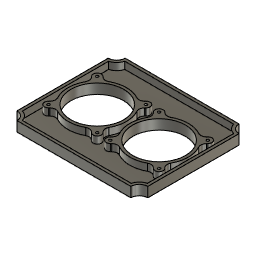
internal_frame (Autodesk Fusion 360 design; units mm, degrees)
Autodesk Fusion 360 part; units mm, degrees
note: some values were not read from the file. Set by a fixed rule: which face or edge a step refers to.
sketch "Sketch1" plane through (0, 0, 0) normal (0, 0, 1) x (1, 0, 0)
  line L0 (69.35, 57.35) -> (-69.35, 57.35)
  line L1 (-69.35, 57.35) -> (-69.35, -57.35)
  line L2 (-69.35, -57.35) -> (69.35, -57.35)
  line L3 (69.35, -57.35) -> (69.35, 57.35)
  line L4 (69.35, 57.35) -> (-69.35, -57.35) construction
  line L5 (-69.35, 57.35) -> (69.35, -57.35) construction
  circle A0 centre (-69.35, -57.35) radius 9
  circle A1 centre (-69.35, 57.35) radius 9
  circle A2 centre (69.35, 57.35) radius 9
  circle A3 centre (69.35, -57.35) radius 9
  line L6 (-69.35, 0) -> (69.35, 0) construction
  line L7 (0, 57.35) -> (0, -57.35) construction
  dimension "d1" = 138.7
  dimension "d2" = 114.7
  dimension "d3" = 18
  dimension "d4" = 18
  dimension "d5" = 18
  dimension "d6" = 18
  constraint horizontal L0
  constraint perpendicular L0 L1
  constraint parallel L0 L2
  constraint parallel L1 L3
  constraint coincident L4 origin
  constraint coincident L5 origin
  constraint coincident L1.end L2.start
  constraint coincident L0.end L1.start
  constraint coincident L0.start L3.end
  constraint coincident L2.end L3.start
  constraint midpoint L1 L6.start
  constraint midpoint L3 L6.end
  constraint midpoint L0 L7.start
  constraint midpoint L2 L7.end
  measures "d1" distance of L1 L3
  measures "d2" distance of L0 L2
  measures "d3" diameter of A0
  measures "d4" diameter of A1
  measures "d5" diameter of A2
  measures "d6" diameter of A3
extrude "Extrude1" add sketch "Sketch1" along normal blind 10.5 contours L0 L1 L2 L3 A0 A1 A2 A3
sketch "Sketch2" plane through (0, 0, 10.5) normal (0, 0, 1) x (-1, 0, 0)
  line L0 (69.35, -48.35) -> (69.35, 48.35)
  arc A0 (60.35, 57.35) -> (69.35, 48.35) centre (69.35, 57.35) ccw
  line L1 (60.35, 57.35) -> (-60.35, 57.35)
  arc A1 (-69.35, 48.35) -> (-60.35, 57.35) centre (-69.35, 57.35) ccw
  line L2 (-69.35, 48.35) -> (-69.35, -48.35)
  arc A2 (-60.35, -57.35) -> (-69.35, -48.35) centre (-69.35, -57.35) ccw
  line L3 (-60.35, -57.35) -> (60.35, -57.35)
  arc A3 (69.35, -48.35) -> (60.35, -57.35) centre (69.35, -57.35) ccw
  line L4 (69.35, 0) -> (-69.8, 0) construction
  line L5 (0, -57.35) -> (0, 57.35) construction
  circle A4 centre (32.6, 0) radius 28
  circle A5 centre (-33, 0) radius 28
  line L6 (-5, -37.1014) -> (-5, 36.8081) construction
  line L7 (4.6, -36.5148) -> (4.6, 40.6209) construction
  line L8 (-61, -35.195) -> (-61, 33.5819) construction
  line L9 (60.6, -36.0749) -> (60.6, 31.9688) construction
  line L10 (53.819, 28) -> (8.2122, 28) construction
  line L11 (-10.8518, 28) -> (-54.5522, 28) construction
  line L12 (6.75, -25.85) -> (58.45, -25.85) construction
  line L13 (58.45, -25.85) -> (58.45, 25.85) construction
  line L14 (58.45, 25.85) -> (6.75, 25.85) construction
  line L15 (6.75, 25.85) -> (6.75, -25.85) construction
  line L16 (6.75, -25.85) -> (58.45, 25.85) construction
  line L17 (58.45, -25.85) -> (6.75, 25.85) construction
  line L18 (-58.85, -25.85) -> (-7.15, -25.85) construction
  line L19 (-7.15, -25.85) -> (-7.15, 25.85) construction
  line L20 (-7.15, 25.85) -> (-58.85, 25.85) construction
  line L21 (-58.85, 25.85) -> (-58.85, -25.85) construction
  line L22 (-58.85, -25.85) -> (-7.15, 25.85) construction
  line L23 (-7.15, -25.85) -> (-58.85, 25.85) construction
  circle A6 centre (58.45, -25.85) radius 1.35
  circle A7 centre (6.75, 25.85) radius 1.35
  circle A8 centre (6.75, -25.85) radius 1.35
  circle A9 centre (-7.15, -25.85) radius 1.35
  circle A10 centre (-7.15, 25.85) radius 1.35
  circle A11 centre (-58.85, 25.85) radius 1.35
  circle A12 centre (-58.85, -25.85) radius 1.35
  circle A13 centre (58.45, 25.85) radius 1.35
  line L24 (-69.35, 30) -> (70.3, 30)
  line L25 (69.35, -30) -> (-69.35, -30)
  line L26 (51.0272, -28) -> (12.0546, -28) construction
  point P0 (32.6, 0)
  point P1 (-33, 0)
  dimension "d9" = 56
  dimension "d10" = 56
  dimension "d11" = 65.6
  dimension "d12" = 9.6
  dimension "d16" = 29.35
  dimension "d17" = 51.7
  dimension "d18" = 51.7
  dimension "d19" = 51.7
  dimension "d20" = 51.7
  dimension "d21" = 2.7
  dimension "d22" = 2.7
  dimension "d23" = 2.7
  dimension "d24" = 2.7
  dimension "d25" = 2.7
  dimension "d26" = 2.7
  dimension "d27" = 2.7
  dimension "d28" = 2.7
  dimension "d31" = 2
  dimension "d32" = 2
  constraint midpoint L0 L4.start
  constraint perpendicular L0 L4
  constraint midpoint L3 L5.start
  constraint midpoint L1 L5.end
  constraint coincident L4 P0
  constraint coincident L4 P1
  constraint perpendicular L4 L6
  constraint tangent A5 L6
  constraint parallel L5 L7
  constraint tangent A4 L7
  constraint vertical L8
  constraint perpendicular L4 L9
  constraint tangent A4 L9
  constraint tangent A5 L8
  constraint perpendicular L7 L10
  constraint horizontal L11
  constraint tangent A4 L10
  constraint tangent A5 L11
  constraint horizontal L12
  constraint perpendicular L12 L13
  constraint parallel L12 L14
  constraint parallel L13 L15
  constraint coincident L16 P0
  constraint coincident L17 P0
  constraint coincident P0 A4.centre
  constraint horizontal L18
  constraint perpendicular L18 L19
  constraint parallel L18 L20
  constraint parallel L19 L21
  constraint coincident L22 P1
  constraint coincident L23 P1
  constraint coincident P1 A5.centre
  constraint coincident L12.end L13.start
  constraint coincident L14.end L15.start
  constraint coincident L12.start L15.end
  constraint coincident L18.end L19.start
  constraint coincident L19.end L20.start
  constraint coincident L20.end L21.start
  constraint coincident L18.start L21.end
  constraint coincident L13.end L14.start
  constraint coincident L2 L24.start
  constraint perpendicular L2 L24
  constraint coincident L0 L25.start
  constraint coincident L2 L25.end
  constraint perpendicular L2 L25
  constraint horizontal L26
  constraint tangent A4 L26
  measures "d9" diameter of A4
  measures "d10" diameter of A5
  measures "d11" distance of P0 P1
  measures "d12" distance of L6 L7
  measures "d16" distance of L1 L11
  measures "d17" distance of L13 L15
  measures "d18" distance of L12 L14
  measures "d19" distance of L19 L21
  measures "d20" distance of L18 L20
  measures "d21" diameter of A6
  measures "d22" diameter of A7
  measures "d23" diameter of A8
  measures "d24" diameter of A9
  measures "d25" diameter of A10
  measures "d26" diameter of A11
  measures "d27" diameter of A12
  measures "d28" diameter of A13
  measures "d31" distance of L11 L24
  measures "d32" distance of L25 L26
extrude "Extrude2" cut sketch "Sketch2" against normal up to surface (10.5 mm away) contours A4 | A5 | A6 | A7 | A8 | A9 | A10 | A11 | A12 | A13
shell "Shell1" thickness 3 removed faces 1 at (-2.25, -47.3, 10.5)
sketch "Sketch3" plane through (0, 0, 10.5) normal (0, 0, 1) x (-1, 0, 0)
  circle A0 centre (58.45, 25.85) radius 4.35
  circle A1 centre (58.45, 25.85) radius 1.35
  line L0 (96.2828, -12.0828) -> (58.4, 25.8)
  line L1 (58.4, 25.8) -> (37.8385, 46.3615)
  line L2 (76.0799, 25.8) -> (20.4357, 25.8) construction
  line L3 (55.3241, 28.8759) -> (49.6672, 23.2191)
  line L4 (61.4759, 22.7241) -> (55.8191, 17.0672)
  line L5 (55.8191, 17.0672) -> (49.6672, 23.2191)
  dimension "d34" = 45
  dimension "d35" = 8
  dimension "d36" = 8
  constraint coincident A0.centre L0.end
  constraint parallel L0 L1
  constraint horizontal L2
  constraint coincident L0.end L2
  constraint coincident A0 L3.start
  constraint coincident L1 L3.start
  constraint coincident A0 L4.start
  constraint coincident L0 L4.start
  measures "d34" angle of L0 L2
  measures "d35" distance of L3.start L3.end
  measures "d36" distance of L4.start L4.end
extrude "Extrude3" add sketch "Sketch3" against normal up to surface (10.5 mm away) contours A0 L3 L4 L5
fillet "Fillet1" radius 6 2 edges at (-51.2275, -24.7793, 6.75) (-57.3793, -18.6275, 6.75)
pattern_circular "C-Pattern1" count 4 over 360 about axis through (-32.6, 0, -2.1) along (0, 0, 1) of "Extrude3", "Fillet1"
sketch "Sketch4" plane through (0, 0, 10.5) normal (0, 0, 1) x (-1, 0, 0)
  circle A0 centre (-7.15, 25.85) radius 4.35
  circle A1 centre (-7.15, 25.85) radius 1.35
  line L0 (-27.2826, 33.6671) -> (20.0548, 33.6671) construction
  line L1 (-7.15, 25.85) -> (-21.4201, 40.1201) construction
  line L2 (-7.15, 25.85) -> (1.607, 17.093) construction
  line L3 (-10.2259, 28.9259) -> (-15.8828, 23.2691)
  line L4 (-4.0741, 22.7741) -> (-9.7309, 17.1172)
  line L5 (-9.7309, 17.1172) -> (-15.8828, 23.2691)
  dimension "d43" = 45
  dimension "d44" = 8
  dimension "d45" = 8
  constraint horizontal L0
  constraint coincident A0.centre A1.centre
  constraint parallel L1 L2
  constraint coincident A0 L3.start
  constraint coincident L1 L3.start
  constraint perpendicular L1 L3
  constraint coincident L2 L4.start
  constraint coincident A0 L4.start
  constraint perpendicular L2 L4
  measures "d43" angle of L0 L1
  measures "d44" distance of L3.start L3.end
  measures "d45" distance of L4.start L4.end
extrude "Extrude4" add sketch "Sketch4" against normal up to surface (7.5 mm away) contours A0 L3 L4 L5
fillet "Fillet2" radius 6 2 edges at (14.3725, -24.7793, 6.75) (8.2207, -18.6275, 6.75)
pattern_circular "C-Pattern2" count 4 over 360 about axis through (33, 0, -2.1) along (0, 0, 1) of "Extrude4", "Fillet2"
